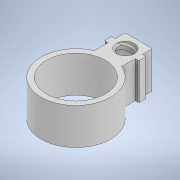
# Autodesk Inventor part: lead_screw_nut
Saved by Autodesk Inventor 2021 (Build 250183000, 183)
## iProperties
Created: 2020-05-25
Part Number: lead_screw_nut
Material: Generic
Document SubType Name: Modeling
Designer: Daniel
Density: 1 g/cm^3
Appearance: Default
Author: Daniel
Autodesk Inventor part; units mm, degrees
ref_plane "YZ Plane" through (0, 0, 0) normal (1, 0, 0) x (0, 1, 0)
ref_plane "XZ Plane" through (0, 0, 0) normal (0, 1, 0) x (-1, 0, 0)
ref_plane "XY Plane" through (0, 0, 0) normal (0, 0, 1) x (1, 0, 0)
sketch "Sketch10" plane through (0, 0, 0) normal (0, 1, 0) x (-1, 0, 0)
  line L0 (7.5, 7.5) -> (-7.5, 7.5)
  line L1 (-7.5, 7.5) -> (-7.5, -7.5)
  line L2 (-7.5, -7.5) -> (7.5, -7.5)
  line L3 (7.5, -7.5) -> (7.5, 7.5)
  line L4 (7.5, 7.5) -> (-7.5, -7.5) construction
  line L5 (-7.5, 7.5) -> (7.5, -7.5) construction
  point P0 (0, 0)
  dimension "d80" = 15
  dimension "d81" = 15
  constraints: 12 end point, 2 midpoint, 2 parallel, 1 horizontal, 1 perpendicular
  measures "d80" distance of L2.end L1.end
  measures "d81" distance of L1.end L0.end
sketch "Sketch11" plane through (0, 0, 0) normal (0, 0, 1) x (1, 0, 0)
  line L0 (0, 0) -> (5, 0) construction
  line L1 (5, 0) -> (5, -20) construction
  line L2 (5, -20) -> (0, -20) construction
  line L3 (0, -20) -> (0, 0) construction
  line L4 (3.851, -20) -> (3.851, 0)
  line L5 (5, -20.75) -> (3.701, -21.5) construction
  line L6 (3.701, -21.5) -> (3.701, -20)
  line L7 (3.701, -20) -> (5, -20.75)
  line L8 (3.851, 0) -> (0, 0)
  line L9 (0, -20) -> (0, 0)
  line L10 (0, -20) -> (3.851, -20)
  line L11 (0, -30.06) -> (0, 5.01) projected
  line L12 (5, -20.75) -> (5, -24.3)
  line L13 (5, -24.3) -> (3.701, -25.05)
  line L14 (3.701, -25.05) -> (3.701, -21.5)
  point P0 (4.134, -20.75)
  point P1 (9.188, -18.332)
  point P2 (0.5278, -18.168)
  dimension "d57" = 10
  dimension "d58" = 20
  dimension "d59" = 1.5
  dimension "d62" = 0.15
  dimension "d77" = 3.55
  constraints: 28 end point, 6 point on line, 4 parallel, 3 perpendicular, 2 collinear, 2 vertical, 1 horizontal, 7 other
  measures "d57" diameter of L1 L3
  measures "d58" distance between parallel lines of L0 L2
  measures "d59" distance of L5.end L6.end
  measures "d62" distance between parallel lines of L6 L4
  measures "d77" distance of L5.start L12.end
extrude "Extrusion7" add sketch "Sketch10" against normal blind 20
revolve "Revolution3" cut sketch "Sketch11" angle 360 about axis through (0, -10, 0) along (0, 1, 0) contours L10 L9 L8 L4
chamfer "Chamfer1" distance 1 angle 45 2 edges at (-3.851, 0, 0) (-3.851, -20, 0)
coil "Coil2" sketch "Sketch11" operation cut axis through (0, -10, 0) along (0, 1, 0) pitch 7 turns 3.857143 hand right contours L7 L12 L13 L14 L6
sketch "Sketch12" plane through (0, 0, 0) normal (0, 1, 0) x (1, 0, 0)
  line L0 (-7.5, -7.5) -> (-7.5, 7.5) projected
  line L1 (7.5, 7.5) -> (7.5, -7.5) projected
  line L2 (5.5, -2) -> (9.5, -2)
  line L3 (9.5, -2) -> (9.5, 2)
  line L4 (9.5, 2) -> (5.5, 2)
  line L5 (5.5, 2) -> (5.5, -2)
  line L6 (5.5, -2) -> (9.5, 2) construction
  line L7 (9.5, -2) -> (5.5, 2) construction
  line L8 (-9.5, -2) -> (-5.5, -2)
  line L9 (-5.5, -2) -> (-5.5, 2)
  line L10 (-5.5, 2) -> (-9.5, 2)
  line L11 (-9.5, 2) -> (-9.5, -2)
  line L12 (-9.5, -2) -> (-5.5, 2) construction
  line L13 (-5.5, -2) -> (-9.5, 2) construction
  point P0 (0, 0)
  point P1 (7.5, 0)
  point P2 (-7.5, 0)
  point P3 (-7.5, -2)
  point P4 (-7.5, 2)
  point P5 (7.5, 2)
  point P6 (7.5, -2)
  dimension "d90" = 4
  dimension "d91" = 4
  dimension "d92" = 4
  dimension "d93" = 4
  constraints: 24 end point, 6 midpoint, 4 parallel, 2 horizontal, 2 perpendicular
  measures "d90" distance of L4.end L3.end
  measures "d91" distance of L3.end L2.end
  measures "d92" distance of L10.end L9.end
  measures "d93" distance of L9.end L8.end
extrude "Extrusion8" add sketch "Sketch12" against normal up to surface (20 mm away) contours L8 L11 L10 L0 | L4 L3 L2 L1
sketch "Sketch13" plane through (0, 0, 0) normal (0, 1, 0) x (1, 0, 0)
  circle A0 centre (0, -27.0659) radius 16.1
  circle A1 centre (0, -27.0659) radius 19.1
  line L0 (-7.5, -7.5) -> (7.5, -7.5) projected
  line L1 (-7.5, -7.5) -> (7.5, -7.5)
  line L2 (7.5, -7.5) -> (7.5, -9.5)
  line L3 (7.5, -9.5) -> (-7.5, -9.5)
  line L4 (-7.5, -9.5) -> (-7.5, -7.5)
  line L5 (7.5, -7.5) -> (7.5, 7.5) projected
  point P0 (0, 0)
  point P1 (7.5, -2)
  dimension "d86" = 32.2
  dimension "d87" = 3
  dimension "d95" = 2
  constraints: 8 end point, 2 centre point, 2 parallel, 2 point on circle, 1 coincident, 1 collinear, 1 horizontal, 1 perpendicular
  measures "d86" diameter of A0
  measures "d87" radial gap between concentric circles of A1 A0
  measures "d95" distance of L3.end L0.start
extrude "Extrusion9" add sketch "Sketch13" against normal up to surface (20 mm away)
fillet "Fillet4" radius 0.5 6 edges at (9.5, -10, -2) (9.5, -10, 2) (-9.5, -10, -2) (-9.5, -10, 2) (7.5, -10, -7.5) (-7.5, -10, -7.5)
equation "\"pitch\" = 7"
equation "\"dia_m\" = 32.2"
body "Solid1"
body "Solid3"
